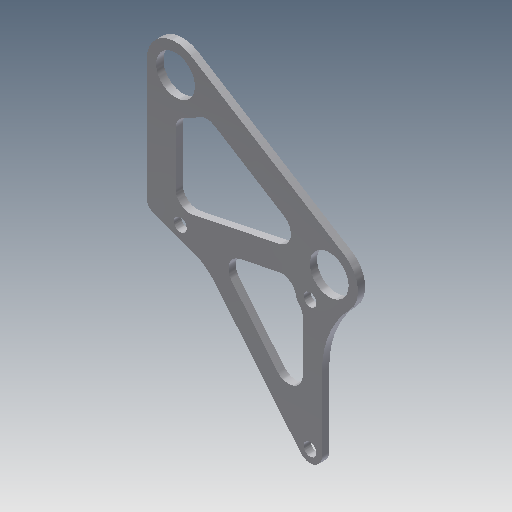
# Autodesk Inventor part: 膝_メインフレーム_1_1
Saved by Autodesk Inventor 2017.3 (Build 213256000, 256)
## iProperties
Created: 2016-04-27
Part Number: 膝_メインフレーム_1_1
Material: アルミニウム 2014-T4
Document SubType Name: Modeling
Designer: hiroaki
Density: 2.8 g/cm^3
Appearance: サテン
Mass: 3.66216 g
Surface Area: 22.9881 cm^2
Volume: 1.30792 cm^3
Author: hiroaki
Autodesk Inventor part; units mm, degrees
ref_plane "YZ Plane" through (0, 0, 0) normal (1, 0, 0) x (0, 1, 0)
ref_plane "XZ Plane" through (0, 0, 0) normal (0, 1, 0) x (-1, 0, 0)
ref_plane "XY Plane" through (0, 0, 0) normal (0, 0, 1) x (1, 0, 0)
derived "下半身全体像_1_1.ipt"
sketch "スケッチ1" plane through (0, 0, 0) normal (0, 0, 1) x (1, 0, 0)
  circle A0 centre (0, 0) radius 10.5 construction
  line L0 (0, 0) -> (-12, 0) construction
  arc A1 (0, 16) -> (-12, 10.583) centre (0, 0) ccw construction
  arc A2 (-12, -10.583) -> (0, -16) centre (0, 0) ccw construction
  line L1 (0, 16) -> (39.5, 16) construction
  line L2 (39.5, 16) -> (39.5, -16) construction
  line L3 (39.5, -16) -> (0, -16) construction
  circle A3 centre (1, 13.5) radius 1.35
  circle A4 centre (1, -13.5) radius 1.35
  circle A5 centre (28, 13.5) radius 1.35
  circle A6 centre (28, -13.5) radius 1.35
  line L4 (1, 13.5) -> (1, -13.5) construction
  line L5 (1, -13.5) -> (28, -13.5) construction
  line L6 (1, 13.5) -> (28, 13.5) construction
  line L7 (28, 13.5) -> (28, -13.5) construction
  line L8 (0, 0) -> (1, 0) construction
  line L9 (32, 120) -> (32, 20) construction
  line L10 (0, 0) -> (0, 0) construction
  circle A7 centre (32, 120) radius 4.05
  line L11 (0, 140) -> (0, 40) construction
  circle A8 centre (0, 40) radius 4.05 construction
  line L12 (0, 0) -> (0, -100) construction
  line L13 (32, 20) -> (32, -80) construction
  line L14 (0, 0) -> (0, 40) construction
  circle A9 centre (32, 20) radius 6.5 construction
  line L15 (32, 23.5218) -> (35.05, 21.7609) construction
  line L16 (35.05, 21.7609) -> (35.05, 18.2391) construction
  line L17 (35.05, 18.2391) -> (32, 16.4782) construction
  line L18 (32, 16.4782) -> (28.95, 18.2391) construction
  line L19 (28.95, 18.2391) -> (28.95, 21.7609) construction
  line L20 (28.95, 21.7609) -> (32, 23.5218) construction
  line L21 (21.5, 152) -> (61, 152) construction
  line L22 (61, 152) -> (61, 100.5) construction
  line L23 (61, 100.5) -> (21.5, 100.5) construction
  line L24 (21.5, 100.5) -> (21.5, 152) construction
  line L25 (21.5, 140) -> (61, 140) construction
  line L26 (16, 150.5) -> (66.5, 150.5) construction
  line L27 (66.5, 150.5) -> (66.5, 129.5) construction
  line L28 (66.5, 129.5) -> (16, 129.5) construction
  line L29 (16, 129.5) -> (16, 150.5) construction
  circle A10 centre (0, 140) radius 10.5 construction
  line L30 (-13.5, 139) -> (13.5, 139) construction
  line L31 (13.5, 139) -> (13.5, 112) construction
  line L32 (13.5, 112) -> (-13.5, 112) construction
  line L33 (-13.5, 112) -> (-13.5, 139) construction
  circle A11 centre (-13.5, 139) radius 1.35
  circle A12 centre (13.5, 139) radius 1.35
  circle A13 centre (-13.5, 112) radius 1.35
  circle A14 centre (13.5, 112) radius 1.35
  line L34 (-12, 10.583) -> (-12, -10.583) construction
  circle A15 centre (0, -100) radius 4.05
  circle A16 centre (32, -80) radius 4.05
  circle A17 centre (0, -100) radius 10.5 construction
  line L35 (32, -80) -> (0, -100) construction
  line L36 (45, -60.5) -> (77.5, -60.5) construction
  line L37 (77.5, -60.5) -> (77.5, -112) construction
  line L38 (77.5, -112) -> (45, -112) construction
  line L39 (45, -112) -> (45, -60.5) construction
  line L40 (45, -100) -> (77.5, -100) construction
  line L41 (39.5, -89.5) -> (83, -89.5) construction
  line L42 (83, -89.5) -> (83, -110.5) construction
  line L43 (83, -110.5) -> (39.5, -110.5) construction
  line L44 (39.5, -110.5) -> (39.5, -89.5) construction
  line L45 (1, -86.5) -> (28, -86.5) construction
  line L46 (28, -86.5) -> (28, -113.5) construction
  line L47 (28, -113.5) -> (1, -113.5) construction
  line L48 (1, -113.5) -> (1, -86.5) construction
  circle A18 centre (1, -86.5) radius 1.35
  circle A19 centre (1, -113.5) radius 1.35
  circle A20 centre (28, -113.5) radius 1.35
  circle A21 centre (28, -86.5) radius 1.35
  circle A22 centre (32, 20) radius 4.05 construction
  circle A23 centre (32, 20) radius 4.05 construction
  line L49 (10.583, 152) -> (-10.583, 152) construction
  line L50 (16, 140) -> (16, 100.5) construction
  line L51 (16, 100.5) -> (-16, 100.5) construction
  line L52 (-16, 100.5) -> (-16, 140) construction
  arc A24 (16, 140) -> (10.583, 152) centre (0, 140) ccw construction
  arc A25 (-10.583, 152) -> (-16, 140) centre (0, 140) ccw construction
  line L53 (-12, -89.417) -> (-12, -110.583) construction
  line L54 (0, -84) -> (39.5, -84) construction
  line L55 (39.5, -84) -> (39.5, -116) construction
  line L56 (39.5, -116) -> (0, -116) construction
  arc A26 (0, -84) -> (-12, -89.417) centre (0, -100) ccw construction
  arc A27 (-12, -110.583) -> (0, -116) centre (0, -100) ccw construction
  circle A28 centre (0, 40) radius 4.05
  line L57 (-6, 40) -> (-6, 13.3451)
  arc A29 (8.1481, 6.7015) -> (3.5479, 9.9355) centre (0, 0) ccw
  circle A30 centre (1, 13.5) radius 2.5 construction
  line L58 (1.7609, 36.95) -> (-1.7609, 36.95) construction
  line L59 (-1.7609, 36.95) -> (-3.5218, 40) construction
  line L60 (-3.5218, 40) -> (-1.7609, 43.05) construction
  line L61 (-1.7609, 43.05) -> (1.7609, 43.05) construction
  line L62 (1.7609, 43.05) -> (3.5218, 40) construction
  line L63 (3.5218, 40) -> (1.7609, 36.95) construction
  circle A31 centre (0, 40) radius 6 construction
  arc A32 (3.18, 45.088) -> (-6, 40) centre (0, 40) ccw
  circle A33 centre (28, -13.5) radius 2.5 construction
  arc A34 (26.0692, -15.088) -> (30.5, -13.5) centre (28, -13.5) ccw
  line L64 (8.1481, 6.7015) -> (26.0692, -15.088)
  line L65 (-6, 13.3451) -> (3.5479, 9.9355)
  circle A35 centre (-8.5, 0) radius 1.35
  circle A36 centre (0, 0) radius 8.5 construction
  line L66 (35.05, 121.7609) -> (35.05, 118.2391) construction
  line L67 (35.05, 118.2391) -> (32, 116.4782) construction
  line L68 (32, 116.4782) -> (28.95, 118.2391) construction
  line L69 (28.95, 118.2391) -> (28.95, 121.7609) construction
  line L70 (28.95, 121.7609) -> (32, 123.5218) construction
  line L71 (32, 123.5218) -> (35.05, 121.7609) construction
  line L72 (0, 152) -> (0, 140) construction
  line L73 (0, 140) -> (0, 139) construction
  line L74 (30.5, -13.5) -> (30.5, 12.0884)
  circle A37 centre (28, 13.5) radius 2.5 construction
  line L75 (3.18, 45.088) -> (35.18, 25.088)
  line L76 (30.5, 12.0884) -> (35.0989, 14.8622)
  arc A38 (35.0989, 14.8622) -> (35.18, 25.088) centre (32, 20) ccw
  circle A39 centre (32, 20) radius 4.05
  point P0 (66.5, 140)
  point P1 (39.5, 0)
  point P2 (83, -100)
  point P3 (1, -100)
  point P4 (-12, -100)
  point P5 (39.5, -100)
  dimension "d4" = 12
  dimension "d1" = 8.1
  dimension "d2" = 10.55
  dimension "d3" = 6.1
  dimension "d48" = 8.1
  dimension "d49" = 6
  measures "d1" diameter of A28
  measures "d2" radius of A29
  measures "d3" distance between parallel lines of L58 L61
  measures "d48" diameter of A39
  measures "d49" radius of A38
extrude "押し出し1" add sketch "スケッチ1" along normal blind 1.5 contours A32 L75 A38 L76 L74 A34 L64 A29 L65 L57
fillet "フィレット1" radius 2 1 edges at (-6, 13.3451, 0.75)
fillet "フィレット1" radius 20 1 edges at (30.5, 12.0884, 0.75)
sketch "スケッチ5" plane through (30.5, -13.5, 1.5) normal (0, 0, 1) x (1, 0, 0)
  line L0 (-22.3519, 20.2015) -> (-4.4308, -1.588) projected
  line L1 (0, 0) -> (0, 25.5884) projected
  arc A0 (-27.32, 58.588) -> (-36.5, 53.5) centre (-30.5, 53.5) ccw projected
  line L2 (-36.5, 53.5) -> (-36.5, 28.2546) projected
  circle A1 centre (-2.5, 27) radius 1.35 projected
  circle A2 centre (-29.5, 27) radius 1.35 projected
  line L3 (-30.5, 46.5) -> (-30.5, 29.3447)
  arc A3 (-30.5, 46.5) -> (-24.564, 49.79) centre (-30.5, 53.5) ccw
  line L4 (-24.564, 49.79) -> (-4.436, 37.21)
  line L5 (-30.5, 29.3447) -> (-5.4122, 34.605)
  arc A4 (-4.436, 37.21) -> (-5.4122, 34.605) centre (1.5, 33.5) ccw
  line L6 (-21.9631, 26.0259) -> (-4, 4.1852)
  line L7 (-4, 4.1852) -> (-4, 24.4019)
  line L8 (-21.9631, 26.0259) -> (-6.0602, 29.3604)
  arc A5 (-5.4362, 26.3844) -> (-4, 24.4019) centre (-2.5, 27) ccw
  line L9 (-6.0602, 29.3604) -> (-5.4362, 26.3844)
  line L10 (4.68, 38.588) -> (-27.32, 58.588) projected
  arc A6 (4.5989, 28.3622) -> (4.68, 38.588) centre (1.5, 33.5) ccw projected
  circle A7 centre (1.5, 33.5) radius 4.05 projected
  line L11 (-29.5, 27) -> (1.5, 33.5) construction
  dimension "d37" = 7
  dimension "d39" = 6
  dimension "d43" = 4
  dimension "d44" = 4
  dimension "d51" = 6
  dimension "d52" = 5
  dimension "d53" = 3
  constraints: 16 end point, 6 point on circle, 5 parallel, 4 coincident, 3 centre point, 1 equal radius, 1 perpendicular, 1 tangent, 1 vertical, 1 other
  measures "d37" radius of A3
  measures "d39" distance between parallel lines of L2 L3
  measures "d43" distance between parallel lines of L1 L7
  measures "d44" distance between parallel lines of L0 L6
  measures "d51" distance between parallel lines of L10 L4
  measures "d52" distance between parallel lines of L8 L5
  measures "d53" radius of A5
extrude "押し出し4" cut sketch "スケッチ5" against normal blind 10 contours A3 L4 A4 L5 L3 | L8 L9 A5 L7 L6
fillet "フィレット2" radius 3 9 edges at (0, 33, 0.75) (5.936, 36.29, 0.75) (26.064, 23.71, 0.75) (25.0878, 21.105, 0.75) (0, 15.8447, 0.75) (8.5369, 12.5259, 0.75) (24.4398, 15.8604, 0.75) (26.5, 10.9019, 0.75) (26.5, -9.3148, 0.75)
equation "\"d39\" = d51"
equation "\"d43\" = d38"
equation "\"d44\" = d43"
equation "\"d38\" = 4"
